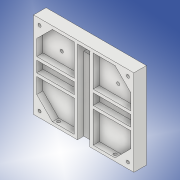
# Autodesk Inventor part: NA002
Saved by Autodesk Inventor 2017 SP1 (Build 210196100, 196)
## iProperties
Created: 2017-06-04
Part Number: NA002
Material: ABS Plastic
Document SubType Name: Modeling
Designer: Zach
Density: 1.06 g/cm^3
Appearance: CR White
Author: Zach
Autodesk Inventor part; units mm, degrees
ref_plane "YZ Plane" through (0, 0, 0) normal (1, 0, 0) x (0, 1, 0)
ref_plane "XZ Plane" through (0, 0, 0) normal (0, 1, 0) x (-1, 0, 0)
ref_plane "XY Plane" through (0, 0, 0) normal (0, 0, 1) x (1, 0, 0)
sketch "Sketch1" plane through (0, 0, 0) normal (0, 0, 1) x (1, 0, 0)
  line L0 (0, 0) -> (160, 0)
  line L1 (160, 0) -> (160, -137.5)
  line L2 (160, -137.5) -> (0, -137.5)
  line L3 (0, -137.5) -> (0, 0)
  dimension "d0" = 160
  dimension "d1" = 137.5
  constraints: 8 end point, 2 parallel, 1 horizontal, 1 perpendicular
  measures "d0" distance of L1.end L2.end
  measures "d1" distance of L0.end L1.end
extrude "Extrusion1" add sketch "Sketch1" along normal blind 10
sketch "Sketch2" plane through (0, 0, 10) normal (0, 0, 1) x (1, 0, 0)
  circle A0 centre (35, -12.5) radius 2.5
  circle A1 centre (35, -37.5) radius 2.5
  line L0 (160, 0) -> (0, 0) projected
  line L1 (0, 0) -> (0, -137.5) projected
  circle A2 centre (125, -12.5) radius 2.5
  circle A3 centre (125, -37.5) radius 2.5
  line L2 (160, -137.5) -> (160, 0) projected
  dimension "d4" = 5
  dimension "d5" = 5
  dimension "d6" = 12.5
  dimension "d7" = 25
  dimension "d8" = 35
  dimension "d9" = 5
  dimension "d10" = 5
  dimension "d11" = 35
  constraints: 4 centre point, 2 horizontal alignment, 2 vertical alignment
  measures "d4" diameter of A0
  measures "d5" diameter of A1
  measures "d6" distance from line of A0.centre L0
  measures "d7" distance of A1.centre A0.centre
  measures "d8" distance from line of L1 A0.centre
  measures "d9" diameter of A2
  measures "d10" diameter of A3
  measures "d11" distance from line of L2 A2.centre
extrude "Extrusion2" cut sketch "Sketch2" against normal through all
sketch "Sketch3" plane through (0, 0, 10) normal (0, 0, 1) x (1, 0, 0)
  circle A0 centre (125, -12.5) radius 2.5 projected
  circle A1 centre (35, -12.5) radius 2.5 projected
  circle A2 centre (35, -37.5) radius 2.5 projected
  circle A3 centre (125, -37.5) radius 2.5 projected
  line L0 (160, 0) -> (0, 0) projected
  line L1 (0, 0) -> (0, -137.5) projected
  line L2 (0, -137.5) -> (160, -137.5) projected
  line L3 (160, -137.5) -> (160, 0) projected
  line L4 (5, -132.5) -> (5, -5)
  line L5 (5, -5) -> (155, -5)
  line L6 (155, -5) -> (155, -132.5)
  line L7 (155, -132.5) -> (5, -132.5)
  dimension "d14" = 5
  constraints: 8 end point, 3 other
  measures "d14" distance between parallel lines of L1 L4
extrude "Extrusion3" add sketch "Sketch3" along normal blind 10 contours L3 L2 L1 L0
sketch "Sketch4" plane through (0, 0, 10) normal (0, 0, 1) x (1, 0, 0)
  line L0 (155, -5) -> (5, -5) projected
  line L1 (70, -5) -> (90, -5)
  line L2 (90, -5) -> (90, -20)
  line L3 (90, -20) -> (70, -20)
  line L4 (70, -20) -> (70, -5)
  line L5 (0, 0) -> (0, -137.5) projected
  dimension "d17" = 20
  dimension "d18" = 15
  dimension "d19" = 70
  constraints: 8 end point, 2 parallel, 1 horizontal, 1 perpendicular, 1 point on line
  measures "d17" distance of L2.end L3.end
  measures "d18" distance of L1.end L2.end
  measures "d19" distance between parallel lines of L5 L4
extrude "Extrusion4" cut sketch "Sketch4" against normal through all
sketch "Sketch5" plane through (5, -132.5, 10) normal (0, 1, 0) x (1, 0, 0)
  circle A0 centre (30, -5) radius 2.5
  circle A1 centre (120, -5) radius 2.5
  line L0 (30, -5) -> (120, -5) construction
  line L1 (-5, -10) -> (155, -10) projected
  point P0 (-5, 10)
  point P1 (75, -10)
  point P2 (75, -5)
  dimension "d22" = 5
  dimension "d23" = 5
  dimension "d24" = 5
  dimension "d25" = 90
  constraints: 2 centre point, 2 end point, 2 midpoint, 1 parallel, 1 vertical alignment
  measures "d22" diameter of A0
  measures "d23" diameter of A1
  measures "d24" distance from line of L1 L0.start
  measures "d25" distance of L0.start L0.end
extrude "Extrusion5" cut sketch "Sketch5" against normal through all
sketch "Sketch6" plane through (5, -132.5, 10) normal (0, 1, 0) x (1, 0, 0)
  line L0 (-5, -10) -> (155, -10) projected
  line L1 (65, -10) -> (85, -10)
  line L2 (85, -10) -> (85, 0)
  line L3 (85, 0) -> (65, 0)
  line L4 (65, 0) -> (65, -10)
  point P0 (-5, 10)
  point P1 (75, -10)
  point P2 (75, -10)
  dimension "d28" = 20
  dimension "d29" = 10
  constraints: 8 end point, 2 midpoint, 2 parallel, 1 coincident, 1 horizontal, 1 perpendicular, 1 point on line
  measures "d28" distance of L3.end L2.end
  measures "d29" distance of L1.end L2.end
extrude "Extrusion6" cut sketch "Sketch6" against normal through all
sketch "Sketch7" plane through (0, 0, 10) normal (0, 0, 1) x (1, 0, 0)
  line L0 (70, -137.5) -> (70, -132.5) projected
  line L1 (70, -132.5) -> (5, -132.5) projected
  line L2 (5, -132.5) -> (5, -5) projected
  line L3 (5, -5) -> (155, -5) projected
  line L4 (155, -5) -> (155, -132.5) projected
  line L5 (155, -132.5) -> (90, -132.5) projected
  line L6 (90, -132.5) -> (90, -137.5) projected
  line L7 (90, -137.5) -> (160, -137.5) projected
  line L8 (160, -137.5) -> (160, 0) projected
  line L9 (160, 0) -> (0, 0) projected
  line L10 (0, 0) -> (0, -137.5) projected
  line L11 (0, -137.5) -> (70, -137.5) projected
  line L12 (5, -132.5) -> (5, -5) projected
  line L13 (5, -55) -> (155, -55)
  line L14 (5, -60) -> (155, -60)
  line L15 (155, -132.5) -> (155, -5) projected
  line L16 (5, -55) -> (5, -60)
  line L17 (155, -55) -> (155, -60)
  line L18 (5, -77.5) -> (155, -77.5)
  line L19 (155, -77.5) -> (155, -82.5)
  line L20 (155, -82.5) -> (5, -82.5)
  line L21 (5, -82.5) -> (5, -77.5)
  dimension "d32" = 5
  dimension "d33" = 50
  dimension "d34" = 5
  dimension "d35" = 50
  constraints: 16 end point, 6 point on line, 2 collinear, 2 horizontal, 2 parallel, 2 perpendicular
  measures "d32" distance of L13.start L14.start
  measures "d33" distance between parallel lines of L3 L13
  measures "d34" distance of L18.end L19.end
  measures "d35" distance between parallel lines of L5 L20
extrude "Extrusion7" add sketch "Sketch7" along normal blind 10 contours L2 L18 L4 L20 | L2 L13 L4 L14
sketch "Sketch8" plane through (0, 0, 10) normal (0, 0, 1) x (1, 0, 0)
  line L0 (90, -5) -> (70, -5) projected
  line L1 (0, -137.5) -> (70, -137.5) projected
  line L2 (70, -5) -> (65, -5)
  line L3 (65, -5) -> (65, -137.5)
  line L4 (65, -137.5) -> (70, -137.5)
  line L5 (70, -137.5) -> (70, -5)
  line L6 (155, -5) -> (90, -5) projected
  line L7 (155, -132.5) -> (90, -132.5) projected
  line L8 (90, -5) -> (95, -5)
  line L9 (95, -5) -> (95, -132.5)
  line L10 (95, -132.5) -> (90, -132.5)
  line L11 (90, -132.5) -> (90, -5)
  point P0 (0, 0)
  dimension "d38" = 5
  dimension "d39" = 5
  constraints: 16 end point, 4 parallel, 2 horizontal, 2 perpendicular, 2 point on line
  measures "d38" distance of L4.end L3.end
  measures "d39" distance of L9.end L10.end
extrude "Extrusion8" add sketch "Sketch8" along normal blind 10
sketch "Sketch9" plane through (0, 0, 10) normal (0, 0, 1) x (1, 0, 0)
  line L0 (90, -137.5) -> (70, -137.5)
  line L1 (70, -137.5) -> (70, -20)
  line L2 (70, -20) -> (90, -20)
  line L3 (90, -20) -> (90, -137.5)
  point P0 (0, 0)
  constraints: 8 end point, 2 parallel, 1 horizontal, 1 perpendicular
extrude "Extrusion9" cut sketch "Sketch9" along normal through all
sketch "Sketch10" plane through (0, 0, 10) normal (0, 0, 1) x (1, 0, 0)
  line L0 (5, -55) -> (5, -5) projected
  line L1 (5, -30) -> (30, -5)
  line L2 (5, -5) -> (65, -5) projected
  line L3 (5, -30) -> (5, -5)
  line L4 (5, -5) -> (30, -5)
  line L5 (155, -5) -> (155, -55) projected
  line L6 (155, -30) -> (130, -5)
  line L7 (95, -5) -> (155, -5) projected
  line L8 (5, -82.5) -> (5, -132.5) projected
  line L9 (5, -132.5) -> (65, -132.5) projected
  line L10 (95, -82.5) -> (95, -132.5) projected
  line L11 (95, -132.5) -> (155, -132.5) projected
  line L12 (155, -132.5) -> (155, -82.5) projected
  line L13 (155, -82.5) -> (95, -82.5) projected
  line L14 (70, -137.5) -> (70, -5) projected
  line L15 (70, -5) -> (90, -5) projected
  line L16 (90, -5) -> (90, -137.5) projected
  line L17 (90, -137.5) -> (160, -137.5) projected
  line L18 (160, -137.5) -> (160, 0) projected
  line L19 (160, 0) -> (0, 0) projected
  line L20 (0, 0) -> (0, -137.5) projected
  line L21 (0, -137.5) -> (70, -137.5) projected
  line L22 (95, -5) -> (155, -5) projected
  line L23 (155, -5) -> (155, -55) projected
  line L24 (155, -55) -> (95, -55) projected
  line L25 (95, -55) -> (95, -5) projected
  line L26 (95, -60) -> (155, -60) projected
  line L27 (155, -60) -> (155, -77.5) projected
  line L28 (155, -77.5) -> (95, -77.5) projected
  line L29 (95, -77.5) -> (95, -60) projected
  line L30 (65, -132.5) -> (5, -132.5) projected
  line L31 (5, -132.5) -> (5, -82.5) projected
  line L32 (65, -60) -> (65, -77.5) projected
  line L33 (65, -77.5) -> (5, -77.5) projected
  line L34 (5, -77.5) -> (5, -60) projected
  line L35 (5, -60) -> (65, -60) projected
  line L36 (95, -132.5) -> (95, -82.5) projected
  line L37 (95, -82.5) -> (155, -82.5) projected
  line L38 (155, -82.5) -> (155, -132.5) projected
  line L39 (155, -132.5) -> (95, -132.5) projected
  line L40 (65, -5) -> (65, -55) projected
  line L41 (65, -55) -> (5, -55) projected
  line L42 (5, -55) -> (5, -5) projected
  line L43 (5, -5) -> (65, -5) projected
  line L44 (130, -5) -> (155, -5)
  line L45 (155, -5) -> (155, -30)
  line L46 (5, -107.5) -> (30, -132.5)
  line L47 (5, -107.5) -> (5, -132.5)
  line L48 (5, -132.5) -> (30, -132.5)
  line L49 (155, -107.5) -> (130, -132.5)
  line L50 (130, -132.5) -> (155, -132.5)
  line L51 (155, -132.5) -> (155, -107.5)
  dimension "d44" = 30
  dimension "d45" = 30
  dimension "d47" = 30
  dimension "d48" = 30
  dimension "d49" = 30
  dimension "d50" = 30
  dimension "d51" = 30
  dimension "d52" = 30
  constraints: 24 end point, 6 collinear, 3 perpendicular, 2 midpoint, 2 point on line
  measures "d44" vertical distance of point (0, 0) L1.start
  measures "d45" horizontal distance of L1.end point (0, 0)
  measures "d47" vertical distance of point (0, 0) L6.start
  measures "d48" horizontal distance of L18.end L6.end
  measures "d49" vertical distance of L20.end L46.start
  measures "d50" horizontal distance of L46.end L20.end
  measures "d51" horizontal distance of L17.end L49.end
  measures "d52" vertical distance of L17.end L49.start
extrude "Extrusion10" add sketch "Sketch10" along normal blind 10 contours L0 L2 L1 | L5 L6 L7 | L46 L9 L8 | L49 L12 L11
sketch "Sketch11" plane through (0, 0, 20) normal (0, 0, 1) x (1, 0, 0)
  circle A0 centre (9.525, -9.525) radius 2.5
  line L0 (0, 0) -> (160, 0) construction
  line L1 (160, 0) -> (160, -137.5) construction
  line L2 (0, 0) -> (160, 0) construction
  line L3 (160, 0) -> (160, -137.5) construction
  line L4 (160, -137.5) -> (0, -137.5) construction
  line L5 (0, -137.5) -> (0, 0) construction
  line L6 (9.525, -9.525) -> (150.475, -9.525) construction
  line L7 (150.475, -9.525) -> (150.475, -127.975) construction
  line L8 (150.475, -127.975) -> (9.525, -127.975) construction
  line L9 (9.525, -127.975) -> (9.525, -9.525) construction
  circle A1 centre (150.475, -9.525) radius 2.5
  circle A2 centre (150.475, -127.975) radius 2.5
  circle A3 centre (9.525, -127.975) radius 2.5
  dimension "d55" = 5
  dimension "d56" = 9.525
  dimension "d57" = 5
  dimension "d58" = 5
  dimension "d59" = 5
  constraints: 16 end point, 4 centre point, 4 coincident, 4 parallel, 2 perpendicular, 1 horizontal, 3 other
  measures "d55" diameter of A0
  measures "d56" distance between parallel lines of L5 L9
  measures "d57" diameter of A1
  measures "d58" diameter of A2
  measures "d59" diameter of A3
extrude "Extrusion11" cut sketch "Sketch11" against normal through all
body "Solid1"
